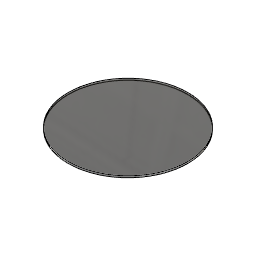
gcan-gauge v31 (Autodesk Fusion 360 archive; units mm, degrees)
design "screen protector 36x0.5mm"
Autodesk Fusion 360 part; units mm, degrees
sketch "Sketch1" plane through (0, 0, 0) normal (0, 0, 1) x (1, 0, 0)
  circle A0 centre (0, 0) radius 18
  dimension "d1" = 36
  constraint coincident A0.centre origin
  measures "d1" diameter of A0
extrude "Extrude1" add sketch "Sketch1" along normal blind 0.5

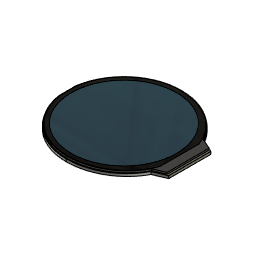
design "lcd"
Autodesk Fusion 360 part; units mm, degrees
sketch "Sketch3" plane through (0, 0, 0) normal (0, 0, 1) x (1, 0, 0)
  line L0 (0, 17.8) -> (0, -17.8) construction
  ellipse E0 centre (0, 0) end of major axis (-17.8, 0) minor radius 17.8 (0, 17.8) -> (0, -17.8) ccw
  line L1 (0, 0) -> (20.3, 0) construction
  line L2 (20.3, 0) -> (20.3, 6.5)
  line L3 (20.3, 6.5) -> (16.4569, 8.1313)
  line L4 (20.3, -6.5) -> (16.4569, -8.1313)
  line L5 (20.3, 0) -> (20.3, -6.5)
  ellipse E1 centre (0, 0) end of major axis (0, 17.8) minor radius 18.5 (0, -17.8) -> (16.4569, -8.1313) ccw
  ellipse E2 centre (0, 0) end of major axis (-0.0369, 17.8) minor radius 18.4985 (16.4569, 8.1313) -> (0, 17.8) ccw
  line L6 (-17.8, 0) -> (-17.8, 7.7502) construction
  dimension "d2" = 35.6
  dimension "d3" = 35.6
  dimension "d4" = 37
  dimension "d5" = 20.3
  dimension "d6" = 6.5
  dimension "d7" = 113
  constraint coincident E0.centre L1.start
  constraint coincident E0.centre L0
  constraint vertical L0
  constraint concentric E0 E1
  constraint horizontal L1
  constraint perpendicular L1 L2
  constraint coincident L3.end E1
  constraint symmetric L2.start L1 L5.start
  constraint symmetric L1 L2.end L4.start
  constraint symmetric L1 L3.end L4.end
  constraint concentric E1 E2
  constraint coincident E0 L6.start
  constraint tangent E0 L6
  constraint perpendicular L1 L6
  measures "d2" distance of E0
  measures "d3" distance of E0
  measures "d5" distance of E0.centre L1.end
  measures "d6" distance of L1.end L2.end
  measures "d7" angle of L2 L3
extrude "Extrude1" add sketch "Sketch3" against normal blind 0.78 makes body 1
sketch "Sketch5" plane through (0, 0, 0) normal (0, 0, 1) x (1, 0, 0)
  line L0 (17.1207, 0) -> (17.1207, 5.9993)
  line L1 (17.1207, 0) -> (17.1207, -5.9993)
  ellipse E0 centre (0, 0) end of major axis (0, 17.3978) minor radius 18.2394 (0, -17.3978) -> (17.1207, -5.9993) ccw
  ellipse E1 centre (0, 0) end of major axis (0, 17.3978) minor radius 18.2394 (17.1207, 5.9993) -> (0, 17.3978) ccw
  line L2 (-17.182, 0) -> (-17.182, 2.542)
  line L3 (-17.182, 0) -> (-17.182, -2.542)
  ellipse E2 centre (0, 0) end of major axis (0, 17.3978) minor radius 17.3684 (0, 17.3978) -> (-17.182, 2.542) ccw
  ellipse E3 centre (0, 0) end of major axis (0, 17.3978) minor radius 17.3684 (-17.182, -2.542) -> (0, -17.3978) ccw
  constraint coincident E0.centre E1.centre
  constraint concentric E0 E2
  constraint coincident L0.end E0
  constraint parallel L0 L1
  constraint concentric E0 E1
  constraint vertical L2
  constraint coincident L3.end E2
  constraint parallel L2 L3
  constraint concentric E2 E3
extrude "Extrude3" add sketch "Sketch5" along normal blind 0.13 separate body makes body 2
sketch "Sketch4" plane through (0, 0, 0.13) normal (0, 0, 1) x (-1, 0, 0)
  line L0 (0, -17.6168) -> (0, 17.6168) construction
  line L1 (-19.7887, 0) -> (-19.7887, -6.4962)
  line L2 (-19.7887, -6.4962) -> (-16.455, -7.9058)
  line L3 (0, 0) -> (-19.7887, 0) construction
  line L4 (-19.7887, 0) -> (-19.7887, 6.4962)
  line L5 (-19.7887, 6.4962) -> (-16.455, 7.9058)
  ellipse E0 centre (0, 0) end of major axis (0, -17.6168) minor radius 18.4133 (-16.455, -7.9058) -> (0, -17.6168) ccw
  ellipse E1 centre (0, 0) end of major axis (0, -17.6168) minor radius 18.4133 (0, 17.6168) -> (-18.4133, 0) ccw
  line L6 (17.4066, 0) -> (17.4066, -2.546)
  line L7 (17.4066, 0) -> (17.4066, 2.546)
  ellipse E2 centre (0, 0) end of major axis (0, -17.6168) minor radius 17.5913 (0, -17.6168) -> (17.4066, -2.546) ccw
  ellipse E3 centre (0, 0) end of major axis (0, -17.6168) minor radius 17.5913 (17.4066, 2.546) -> (0, 17.6168) ccw
  line L8 (17.182, -2.542) -> (17.182, 2.542)
  ellipse E4 centre (0, 0) end of major axis (0, -17.3978) minor radius 17.3684 (17.182, 2.542) -> (0, 17.3978) ccw
  ellipse E5 centre (0, 0) end of major axis (18.2394, 0) minor radius 17.3978 (0, 17.3978) -> (-17.1207, 5.9993) ccw
  line L9 (-17.1207, 5.9993) -> (-17.1207, -5.9993)
  ellipse E6 centre (0, 0) end of major axis (18.2394, 0) minor radius 17.3978 (-17.1207, -5.9993) -> (0, -17.3978) ccw
  ellipse E7 centre (0, 0) end of major axis (0, -17.3978) minor radius 17.3684 (0, -17.3978) -> (17.182, -2.542) ccw
  constraint coincident L3.start E0.centre
  constraint concentric E0 E2
  constraint coincident L0.end E0
  constraint perpendicular L1 L3
  constraint symmetric L1.start L3 L4.start
  constraint symmetric L1.end L3 L4.end
  constraint symmetric L2.end L3 L5.end
  constraint concentric E0 E1
  constraint vertical L6
  constraint coincident L7.end E2
  constraint parallel L6 L7
  constraint concentric E2 E3
extrude "Extrude4" add sketch "Sketch4" along normal blind 0.5 separate body contours L1 L2 L4 L5 E0 E1 L6 L7 E2 E3 | L8 E4 E5 L9 E6 E7 makes body 3
sketch "Sketch6" plane through (0, 0, 0.63) normal (0, 0, 1) x (-1, 0, 0)
  line L0 (17.4066, -2.546) -> (17.4066, 2.546)
  ellipse E0 centre (0, 0) end of major axis (0, -17.6168) minor radius 17.5913 (17.4066, 2.546) -> (0, 17.6168) ccw
  ellipse E1 centre (0, 0) end of major axis (18.4133, 0) minor radius 17.6168 (0, 17.6168) -> (-16.455, 7.9058) ccw
  line L1 (-16.455, 7.9058) -> (-19.7887, 6.4962)
  line L2 (-19.7887, 6.4962) -> (-19.7887, -6.4962)
  line L3 (-19.7887, -6.4962) -> (-16.455, -7.9058)
  ellipse E2 centre (0, 0) end of major axis (18.4133, 0) minor radius 17.6168 (-16.455, -7.9058) -> (0, -17.6168) ccw
  ellipse E3 centre (0, 0) end of major axis (0, -17.6168) minor radius 17.5913 (0, -17.6168) -> (17.4066, -2.546) ccw
  ellipse E4 centre (0, 0) end of major axis (0, -17.3978) minor radius 17.3684 (0, -17.3978) -> (17.182, -2.542) ccw
  ellipse E5 centre (0, 0) end of major axis (18.2394, 0) minor radius 17.3978 (-17.1207, -5.9993) -> (0, -17.3978) ccw
  line L4 (-17.1207, -5.9993) -> (-17.1207, 5.9993)
  ellipse E6 centre (0, 0) end of major axis (18.2394, 0) minor radius 17.3978 (0, 17.3978) -> (-17.1207, 5.9993) ccw
  ellipse E7 centre (0, 0) end of major axis (0, -17.3978) minor radius 17.3684 (17.182, 2.542) -> (0, 17.3978) ccw
  line L5 (17.182, -2.542) -> (17.182, 2.542)
extrude "Extrude5" add sketch "Sketch6" along normal blind 0.09 separate body contours E4 E5 L4 E6 E7 L5 makes body 4
sketch "Sketch7" plane through (0, 0, 0.72) normal (0, 0, 1) x (-1, 0, 0)
  ellipse E0 centre (0, 0) end of major axis (18.2394, 0) minor radius 17.3978 (-17.1207, -5.9993) -> (0, -17.3978) ccw
  ellipse E1 centre (0, 0) end of major axis (0, -17.3978) minor radius 17.3684 (0, -17.3978) -> (17.182, -2.542) ccw
  line L0 (17.182, -2.542) -> (17.182, 2.542)
  ellipse E2 centre (0, 0) end of major axis (0, -17.3978) minor radius 17.3684 (17.182, 2.542) -> (0, 17.3978) ccw
  ellipse E3 centre (0, 0) end of major axis (18.2394, 0) minor radius 17.3978 (0, 17.3978) -> (-17.1207, 5.9993) ccw
  line L1 (-17.1207, 5.9993) -> (-17.1207, -5.9993)
  circle A0 centre (0, 0) radius 16.25
  dimension "d23" = 32.5
  constraint coincident E0.centre E1.centre
  measures "d23" diameter of A0
extrude "Extrude6" cut sketch "Sketch7" against normal blind 0.1 contours A0 bodies 3 4
extrude "Extrude7" add 1 faces at (0.5806, -4.2349, 0.62) along direction (0, 0, 1) blind 0.1 separate body on bodies 3 makes body 5
sketch "Sketch8" plane through (0, 0, -0.78) normal (0, 0, -1) x (1, 0, 0)
  line L0 (20.3, -6.5) -> (20.3, 6.5)
  line L1 (20.3, 6.5) -> (16.4569, 8.1313)
  ellipse E0 centre (0, 0) end of major axis (-18.5, 0) minor radius 17.8 (16.4569, 8.1313) -> (0, 17.8) ccw
  arc A0 (0, 17.8) -> (0, -17.8) centre (0, 0) ccw
  ellipse E1 centre (0, 0) end of major axis (-18.4984, 0.0383) minor radius 17.8 (0, -17.8) -> (16.4569, -8.1313) ccw
  line L2 (16.4569, -8.1313) -> (20.3, -6.5)
  circle A1 centre (0, 0) radius 16.25
sketch "Sketch9" plane through (0, 0, -0.78) normal (0, 0, -1) x (1, 0, 0)
  line L0 (20.3, -6.5) -> (20.3, 6.5)
  line L1 (20.3, 6.5) -> (16.4569, 8.1313)
  ellipse E0 centre (0, 0) end of major axis (-18.5, 0) minor radius 17.8 (16.4569, 8.1313) -> (0, 17.8) ccw construction
  arc A0 (0, 17.8) -> (0, -17.8) centre (0, 0) ccw construction
  ellipse E1 centre (0, 0) end of major axis (-18.4984, 0.0383) minor radius 17.8 (0, -17.8) -> (16.4569, -8.1313) ccw construction
  line L2 (16.4569, -8.1313) -> (20.3, -6.5)
  line L3 (20.3, -6.5) -> (16.4569, -8.1313) construction
  ellipse E2 centre (0, 0) end of major axis (-18.4984, 0.0383) minor radius 17.8 (0, -17.8) -> (16.4569, -8.1313) ccw
  arc A1 (0, 17.8) -> (0, -17.8) centre (0, 0) ccw construction
  ellipse E3 centre (0, 0) end of major axis (-18.5, 0) minor radius 17.8 (16.4569, 8.1313) -> (0, 17.8) ccw
  line L4 (20.3, 6.5) -> (16.4569, 8.1313) construction
  line L5 (20.3, 6.5) -> (20.3, -6.5) construction
  line L6 (0, 0) -> (20.3, 0) construction
  line L7 (16.4569, 8.1313) -> (14.7637, 10.7264)
  line L8 (14.7637, 10.7264) -> (12.1136, 13.4535)
  line L9 (12.1136, 13.4535) -> (8.9838, 15.5603)
  line L10 (8.9838, 15.5603) -> (5.5201, 16.9891)
  line L11 (5.5201, 16.9891) -> (1.8614, 17.7097)
  line L12 (1.8614, 17.7097) -> (-1.8606, 17.7025)
  line L13 (-1.8606, 17.7025) -> (-5.5005, 16.9288)
  line L14 (-5.5005, 16.9288) -> (-8.9, 15.4153)
  line L15 (-8.9, 15.4153) -> (-11.9105, 13.228)
  line L16 (-11.9105, 13.228) -> (-14.4005, 10.4626)
  line L17 (-14.4005, 10.4626) -> (-16.2611, 7.2399)
  line L18 (-16.2611, 7.2399) -> (-17.411, 3.7008)
  line L19 (-17.411, 3.7008) -> (-17.8, 0)
  line L20 (-17.8, 0) -> (-17.411, -3.7008)
  line L21 (-17.411, -3.7008) -> (-16.2611, -7.2399)
  line L22 (-16.2611, -7.2399) -> (-14.4005, -10.4626)
  line L23 (-14.4005, -10.4626) -> (-11.9105, -13.228)
  line L24 (-11.9105, -13.228) -> (-8.9, -15.4153)
  line L25 (-8.9, -15.4153) -> (-5.5005, -16.9288)
  line L26 (-5.5005, -16.9288) -> (-1.8606, -17.7025)
  line L27 (-1.8606, -17.7025) -> (1.8614, -17.7099)
  line L28 (1.8614, -17.7099) -> (5.5203, -16.9898)
  line L29 (5.5203, -16.9898) -> (8.9842, -15.5611)
  line L30 (8.9842, -15.5611) -> (12.1141, -13.4541)
  line L31 (12.1141, -13.4541) -> (14.764, -10.7267)
  line L32 (14.764, -10.7267) -> (16.4569, -8.1313)
  constraint coincident E0.centre A0.centre
  constraint horizontal L6
  constraint coincident L1.end L4.end
  constraint coincident E3 L7.end
  constraint coincident E3 L8.end
  constraint coincident E3 L9.end
  constraint coincident E3 L10.end
  constraint coincident E3 L11.end
  constraint coincident A0 L12.end
  constraint coincident A0 L13.end
  constraint coincident A1 L14.end
  constraint coincident A1 L15.end
  constraint coincident A0 L16.end
  constraint coincident A1 L17.end
  constraint coincident A0 L18.end
  constraint midpoint A1 L19.end
  constraint coincident A0 L20.end
  constraint coincident A1 L21.end
  constraint coincident A0 L22.end
  constraint coincident A0 L23.end
  constraint coincident A1 L24.end
  constraint coincident A0 L25.end
  constraint coincident A0 L26.end
  constraint coincident E2 L27.end
  constraint coincident E2 L28.end
  constraint coincident E2 L29.end
  constraint coincident E2 L30.end
  constraint coincident E2 L31.end
  constraint coincident L2.start L3.end
  constraint coincident L0 L6.end
named bodies: "backlight", "polarizer", "LCD", "front glass"
